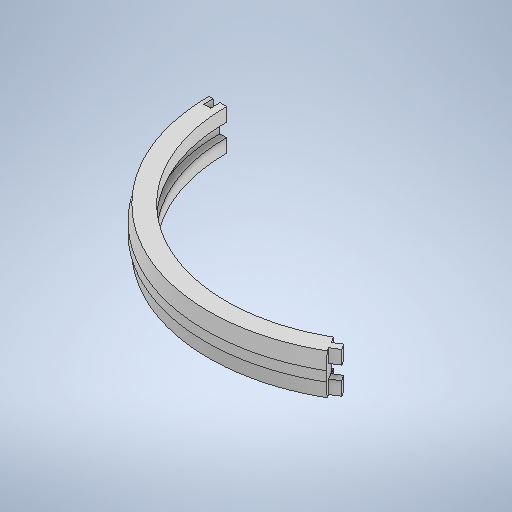
# Autodesk Inventor part: Inner_ring
Saved by Autodesk Inventor 2025 (Build 290162000, 162)
## iProperties
Created: 2025-09-25
Part Number: Inner_ring
Material: Типовые
Document SubType Name: Modeling
Designer: Admin
Density: 1 g/cm^3
Appearance: По умолчанию
Author: Admin
Autodesk Inventor part; units mm, degrees
ref_plane "YZ Plane" through (0, 0, 0) normal (1, 0, 0) x (0, 1, 0)
ref_plane "XZ Plane" through (0, 0, 0) normal (0, 1, 0) x (-1, 0, 0)
ref_plane "XY Plane" through (0, 0, 0) normal (0, 0, 1) x (1, 0, 0)
sketch "Эскиз1" plane through (0, 0, 0) normal (0, 1, 0) x (-1, 0, 0)
  line L0 (0, 0) -> (140, 0)
  line L1 (0, 0) -> (-70, 121.2436)
  line L2 (0, 0) -> (140, 0) construction
  arc A0 (140, 0) -> (-70, 121.2436) centre (0, 0) ccw
  arc A1 (125, 0) -> (-62.5, 108.2532) centre (0, 0) ccw
  line L3 (125, 0) -> (130, 0)
  arc A2 (130, 0) -> (129.8218, 6.8037) centre (0, 0) ccw
  line L4 (0, 0) -> (129.8218, 6.8037) construction
  line L5 (0, 0) -> (130, 0) construction
  line L6 (130, 0) -> (135, 0)
  arc A3 (135, 0) -> (134.815, 7.0654) centre (0, 0) ccw
  line L7 (0, 0) -> (134.815, 7.0654) construction
  line L8 (0, 0) -> (135, 0) construction
  line L9 (134.815, 7.0654) -> (129.8218, 6.8037)
  line L10 (-62.5, 108.2532) -> (-65, 112.5833)
  line L11 (-65, 112.5833) -> (-67.5, 116.9134)
  arc A4 (-65, 112.5833) -> (-70.8031, 109.0272) centre (0, 0) ccw
  line L12 (0, 0) -> (-70.8031, 109.0272) construction
  line L13 (0, 0) -> (-65, 112.5833) construction
  arc A5 (-67.5, 116.9134) -> (-73.5263, 113.2205) centre (0, 0) ccw
  line L14 (0, 0) -> (-73.5263, 113.2205) construction
  line L15 (0, 0) -> (-67.5, 116.9134) construction
  line L16 (-73.5263, 113.2205) -> (-70.8031, 109.0272)
  dimension "d2" = 140
  dimension "d3" = 120
  dimension "d4" = 125
  dimension "d5" = 5
  dimension "d8" = 3
  dimension "d9" = 5
  dimension "d10" = 3
  dimension "d11" = 5
  dimension "d12" = 5
  dimension "d13" = 3
  dimension "d14" = 3
  constraints: 34 end point, 12 point on circle, 6 centre point, 6 coincident, 6 point on line, 2 collinear, 2 horizontal, 1 equal length
  measures "d2" distance of L0.start L1.end
  measures "d3" angle of L2 L1
  measures "d4" radius of A1
  measures "d5" distance of L3.start L3.end
  measures "d8" angle of L5 L4
  measures "d9" distance of L3.end L6.end
  measures "d10" angle of L8 L7
  measures "d11" distance of L10.start L10.end
  measures "d12" distance of L10.end L11.end
  measures "d13" angle of L13 L12
  measures "d14" angle of L15 L14
extrude "Выдавливание1" add sketch "Эскиз1" along normal blind 10 contours A1 L1 A0 L0 A3 L9 A2 | A4 L16 A5 L1
extrude "Выдавливание2" add sketch "Эскиз1" against normal blind 20 contours A1 L1 A0 L0 A3 L9 A2 | A2 L9 A3 L0 | A4 L16 A5 L1
extrude "Выдавливание3" cut sketch "Эскиз1" against normal blind 10 contours A4 L16 A5 L1
extrude "Выдавливание4" cut sketch "Эскиз1" along normal blind 10 and the other way blind 20 contours A2 L9 A3 L0
extrude "Выдавливание5" add sketch "Эскиз1" against normal blind 10 contours A2 L9 A3 L0
chamfer "Фаска1" distance 2 angle 80 1 edges at (-70, 10, 121.2436) measured on face at (-69.75, 10, 120.8105)
chamfer "Фаска2" distance 2 angle 80 1 edges at (-70, -20, 121.2436) measured on face at (-69.75, -20, 120.8105)
sketch "Эскиз2" plane through (0, 10, 0) normal (0, 1, 0) x (1, 0, 0)
  line L0 (65, -112.5833) -> (62.5, -108.2532) projected
  arc A0 (-125, 0) -> (62.5, -108.2532) centre (0, 0) ccw
  arc A1 (65, -112.5833) -> (70.8031, -109.0272) centre (0, 0) ccw projected
  line L1 (-130, 0) -> (-125, 0) projected
  line L2 (65, -112.5833) -> (67.5, -116.9134) projected
  arc A2 (-130, 0) -> (65, -112.5833) centre (0, 0) ccw
  line L3 (-130, 0) -> (-125, 0)
  line L4 (62.5, -108.2532) -> (65, -112.5833)
  constraints: 4 end point, 4 point on circle, 2 centre point, 2 coincident, 1 collinear
extrude "Выдавливание6" cut sketch "Эскиз2" against normal blind 20
extrude "Выдавливание7" add sketch "Эскиз2" against normal blind 10
